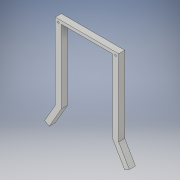
# Autodesk Inventor part: U-Part Gen 2
Saved by Autodesk Inventor 2019 (Build 230136000, 136)
## iProperties
Created: 2019-10-05
Part Number: U-Part Gen 2
Material: Generic
Document SubType Name: Modeling
Designer: Delta
Density: 1 g/cm^3
Appearance: Default
Author: Delta
Autodesk Inventor part; units mm, degrees
ref_plane "YZ Plane" through (0, 0, 0) normal (1, 0, 0) x (0, 1, 0)
ref_plane "XZ Plane" through (0, 0, 0) normal (0, 1, 0) x (-1, 0, 0)
ref_plane "XY Plane" through (0, 0, 0) normal (0, 0, 1) x (1, 0, 0)
sketch "Sketch1" plane through (0, 0, 0) normal (0, 0, 1) x (1, 0, 0)
  line L0 (0, 0) -> (132.08, 0)
  line L1 (132.08, 0) -> (132.08, -6.35)
  line L2 (132.08, -6.35) -> (0, -6.35)
  line L3 (0, -6.35) -> (0, 0)
  line L4 (132.08, 0) -> (119.38, 0)
  line L5 (119.38, 0) -> (119.38, -159.2059)
  line L6 (119.38, -159.2059) -> (132.08, -159.2059)
  line L7 (132.08, -159.2059) -> (132.08, 0)
  line L8 (0, 0) -> (12.7, 0)
  line L9 (12.7, 0) -> (12.7, -159.2059)
  line L10 (12.7, -159.2059) -> (0, -159.2059)
  line L11 (0, -159.2059) -> (0, 0)
  line L12 (0, -146.5059) -> (25.4, -146.5059) construction
  line L13 (12.7, -159.2059) -> (38.1, -159.2059) construction
  line L14 (0, -159.2059) -> (-22.225, -197.7007)
  line L15 (12.7, -159.2059) -> (-12.7, -203.2)
  line L16 (-22.225, -197.7007) -> (-12.7, -203.2)
  line L17 (66.04, 0) -> (66.04, -59.745)
  line L18 (132.08, -159.2059) -> (154.305, -197.7007)
  line L19 (119.38, -159.2059) -> (144.78, -203.2)
  line L20 (154.305, -197.7007) -> (144.78, -203.2)
  dimension "d1" = 6.35
  dimension "d2" = 12.7
  dimension "d3" = 159.2059
  dimension "d5" = 159.2059
  dimension "d6" = 12.7
  dimension "d13" = 12.7
  dimension "d15" = 106.68
  dimension "d28" = 0
  dimension "d29" = 60
  dimension "d30" = 50.8
  dimension "d31" = 53.34
  dimension "d32" = 203.2
  dimension "d33" = 43.9941
  constraints: 42 end point, 6 parallel, 5 horizontal, 4 perpendicular, 2 symmetric about line, 1 midpoint, 1 point on line, 1 vertical
  measures "d1" distance of L0.end L1.end
  measures "d2" distance of L6.end L5.end
  measures "d3" distance of L5.end L4.end
  measures "d5" distance between parallel lines of L10 L0
  measures "d6" distance of L12.start L10.end
  measures "d13" distance between parallel lines of L11 L9
  measures "d15" distance between parallel lines of L5 L9
  measures "d28" angle of L14 L15
  measures "d29" angle of L10 L15
  measures "d30" distance from line of L9.end L16
  measures "d31" distance between parallel lines of L5 L17
  measures "d32" distance from line of L0 L15.end
  measures "d33" distance from line of L10 L15.end
extrude "Extrusion2" add sketch "Sketch1" along normal blind 12.7
sketch "Sketch3" plane through (0, 0, 12.7) normal (0, 0, 1) x (1, 0, 0)
  line L0 (0, 0) -> (0, -159.2059) projected
  line L1 (12.7, -159.2059) -> (12.7, -6.35) projected
  line L2 (132.08, 0) -> (0, 0) projected
  line L3 (132.08, -159.2059) -> (132.08, 0) projected
  circle A0 centre (6.35, -6.35) radius 1.778
  circle A1 centre (125.73, -6.35) radius 1.778
  dimension "d18" = 6.35
  dimension "d19" = 12.7
  dimension "d20" = 6.35
  dimension "d21" = 6.35
  dimension "d22" = 6.35
  dimension "d23" = 3.556
  dimension "d24" = 3.556
  constraints: 2 centre point, 2 coincident
  measures "d18" distance from line of L0 point (6.35, -6.35)
  measures "d19" distance between parallel lines of L0 L1
  measures "d20" distance from line of L2 point (6.35, -6.35)
  measures "d21" distance from line of L2 point (125.73, -6.35)
  measures "d22" distance from line of L3 point (125.73, -6.35)
  measures "d23" diameter of A0
  measures "d24" diameter of A1
extrude "Extrusion3" cut sketch "Sketch3" against normal blind 25.4
equation "\"d3\" = d5"
equation "\"d6\" = d4"
equation "\"d18\" = 0.5 * d19"
equation "\"d21\" = d20"
equation "\"d22\" = d18"
equation "\"d4\" = d2"
body "Solid2"
